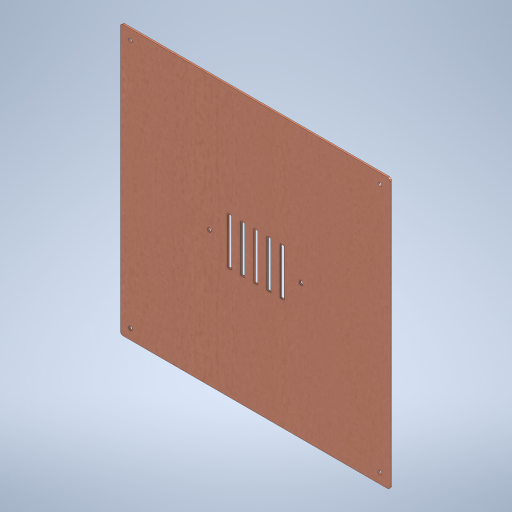
# Autodesk Inventor part: Tapadera
Saved by Autodesk Inventor 2024 (Build 280153000, 153)
## iProperties
Created: 2024-07-17
Part Number: Tapadera
Material: Genérico
Document SubType Name: Modeling
Designer: sergi
Density: 1 g/cm^3
Appearance: Valor por defecto
Author: sergi
Autodesk Inventor part; units mm, degrees
ref_plane "YZ Plane" through (0, 0, 0) normal (1, 0, 0) x (0, 1, 0)
ref_plane "XZ Plane" through (0, 0, 0) normal (0, 1, 0) x (-1, 0, 0)
ref_plane "XY Plane" through (0, 0, 0) normal (0, 0, 1) x (1, 0, 0)
sketch "Boceto1" plane through (0, 0, 0) normal (0, 0, 1) x (1, 0, 0)
  line L0 (-198, 0) -> (0, 0) projected
  line L1 (-198, 0) -> (-198, -2) projected
  line L2 (0, -2) -> (-198, -2) projected
  line L3 (0, 0) -> (0, -2) projected
  line L4 (0, -2) -> (0, -200) projected
  line L5 (0, -2) -> (-2, -2) projected
  line L6 (-2, -200) -> (-2, -2) projected
  line L7 (0, -200) -> (-2, -200) projected
  line L8 (-2, -200) -> (-200, -200) projected
  line L9 (-2, -200) -> (-2, -198) projected
  line L10 (-200, -198) -> (-2, -198) projected
  line L11 (-200, -200) -> (-200, -198) projected
  line L12 (-200, -198) -> (-200, 0) projected
  line L13 (-200, -198) -> (-198, -198) projected
  line L14 (-198, 0) -> (-198, -198) projected
  line L15 (-200, 0) -> (-198, 0) projected
  line L16 (0, 0) -> (0, 1.6)
  line L17 (0, 1.6) -> (1.6, 1.6)
  line L18 (1.6, 1.6) -> (-201.6, 1.6)
  line L19 (-201.6, 1.6) -> (-201.6, -201.6)
  line L20 (-201.6, -201.6) -> (1.6, -201.6)
  line L21 (1.6, -201.6) -> (1.6, 1.6)
  line L22 (-203, 1) -> (-203, -201) projected
  line L23 (-201, -203) -> (1, -203) projected
  line L24 (3, -201) -> (3, 1) projected
  line L25 (1, 3) -> (-201, 3) projected
  line L26 (-192.75, -7.25) -> (-7.25, -7.25) projected
  line L27 (-7.25, -7.25) -> (-7.25, -192.75) projected
  line L28 (-7.25, -192.75) -> (-192.75, -192.75) projected
  line L29 (-192.75, -192.75) -> (-192.75, -7.25) projected
  circle A0 centre (-195.25, -4.75) radius 2.1 projected
  circle A1 centre (-4.75, -4.75) radius 2.1 projected
  circle A2 centre (-4.75, -195.25) radius 2.1 projected
  circle A3 centre (-195.25, -195.25) radius 2.1 projected
  arc A4 (-201, 3) -> (-203, 1) centre (-201, 1) ccw projected
  arc A5 (-203, -201) -> (-201, -203) centre (-201, -201) ccw projected
  arc A6 (1, -203) -> (3, -201) centre (1, -201) ccw projected
  arc A7 (3, 1) -> (1, 3) centre (1, 1) ccw projected
  dimension "d0" = 1.6
  dimension "d1" = 1.6
  dimension "d2" = 203.2
  dimension "d3" = 203.2
  constraints: 12 end point, 2 parallel, 2 perpendicular, 1 horizontal, 1 point on line
  measures "d0" distance of L0.end L16.end
  measures "d1" distance of L16.end L17.end
  measures "d2" distance of L20.end L19.end
  measures "d3" distance of L19.end L18.end
extrude "Extrusión1" add sketch "Boceto1" along normal blind 1.2 contours L17 L21 L20 L19 L18 | L0 L3 L2 L1 | L1 L14 L10 L12 L15 | L2 L6 L10 L14 | L4 L7 L6 L2 | L10 L6 L8 L11 | A4 L25 A7 L24 A6 L23 A5 L22 | L26 L27 L28 L29 | A0 | A1 | A2 | A3
sketch "Boceto2" plane through (0, 0, 1.2) normal (0, 0, 1) x (1, 0, 0)
  line L0 (-192.75, -7.25) -> (-7.25, -7.25) projected
  line L1 (-7.25, -7.25) -> (-7.25, -192.75) projected
  line L2 (-2.25, -197.75) -> (-2.25, -2.25) projected
  line L3 (-2.25, -2.25) -> (-197.75, -2.25) projected
  line L4 (-7.25, -7.25) -> (-2.25, -2.25)
  circle A0 centre (-4.75, -4.75) radius 1.5
  line L5 (-201, -203) -> (1, -203) projected
  line L6 (-203, -203) -> (-203, -195.25)
  line L7 (-203, 1) -> (-203, -201) projected
  line L8 (-203, -195.25) -> (-195.25, -195.25)
  circle A1 centre (-195.25, -195.25) radius 1.5
  line L9 (3, -203) -> (-4.75, -203)
  line L10 (-4.75, -203) -> (-4.75, -195.25)
  circle A2 centre (-4.75, -195.25) radius 1.5
  line L11 (-203, 3) -> (-195.25, 3)
  line L12 (1, 3) -> (-201, 3) projected
  line L13 (-195.25, 3) -> (-195.25, -4.75)
  circle A3 centre (-195.25, -4.75) radius 1.5
  point P0 (0, 0)
  point P1 (3, 3)
  dimension "d6" = 3
  dimension "d14" = 7.75
  dimension "d15" = 7.75
  dimension "d16" = 3
  dimension "d17" = 7.75
  dimension "d18" = 7.75
  dimension "d19" = 3
  dimension "d20" = 7.75
  dimension "d21" = 7.75
  dimension "d22" = 90
  dimension "d23" = 3
  constraints: 14 end point, 4 centre point, 3 coincident, 3 perpendicular, 3 point on line, 1 midpoint
  measures "d6" diameter of A0
  measures "d14" distance of L6.start L6.end
  measures "d15" distance of L6.end L8.end
  measures "d16" diameter of A1
  measures "d17" distance of L9.start L9.end
  measures "d18" distance of L9.end L10.end
  measures "d19" diameter of A2
  measures "d20" distance of L11.start L11.end
  measures "d21" distance of L11.end L13.end
  measures "d22" angle of L11 L13
  measures "d23" diameter of A3
hole "Agujero1" at (-4.75, -4.75, 1.2) at (-195.25, -4.75, 1.2) at (-195.25, -195.25, 1.2) at (-4.75, -195.25, 1.2) direction (0, 0, -1) diameter 3 depth 4
sketch "Boceto3" plane through (0, 0, 1.2) normal (0, 0, 1) x (1, 0, 0)
  line L0 (-125, -122.5) -> (-75, -122.5) projected
  arc A0 (-75, -122.5) -> (-70, -117.5) centre (-75, -117.5) ccw projected
  line L1 (-70, -117.5) -> (-70, -112.2474) projected
  arc A1 (-64, -104.899) -> (-70, -112.2474) centre (-62.5, -112.2474) ccw projected
  arc A2 (-64, -104.899) -> (-64, -95.101) centre (-65, -100) ccw projected
  arc A3 (-70, -87.7526) -> (-64, -95.101) centre (-62.5, -87.7526) ccw projected
  line L2 (-70, -87.7526) -> (-70, -82.5) projected
  arc A4 (-70, -82.5) -> (-75, -77.5) centre (-75, -82.5) ccw projected
  line L3 (-75, -77.5) -> (-125, -77.5) projected
  arc A5 (-125, -77.5) -> (-130, -82.5) centre (-125, -82.5) ccw projected
  line L4 (-130, -82.5) -> (-130, -87.7526) projected
  arc A6 (-136, -95.101) -> (-130, -87.7526) centre (-137.5, -87.7526) ccw projected
  arc A7 (-136, -95.101) -> (-136, -104.899) centre (-135, -100) ccw projected
  arc A8 (-130, -112.2474) -> (-136, -104.899) centre (-137.5, -112.2474) ccw projected
  line L5 (-130, -112.2474) -> (-130, -117.5) projected
  arc A9 (-130, -117.5) -> (-125, -122.5) centre (-125, -117.5) ccw projected
  line L6 (-125, -121.5) -> (-75, -121.5) projected
  arc A10 (-75, -121.5) -> (-71, -117.5) centre (-75, -117.5) ccw projected
  line L7 (-71, -117.5) -> (-71, -82.5) projected
  arc A11 (-71, -82.5) -> (-75, -78.5) centre (-75, -82.5) ccw projected
  line L8 (-75, -78.5) -> (-125, -78.5) projected
  arc A12 (-125, -78.5) -> (-129, -82.5) centre (-125, -82.5) ccw projected
  line L9 (-129, -82.5) -> (-129, -117.5) projected
  arc A13 (-129, -117.5) -> (-125, -121.5) centre (-125, -117.5) ccw projected
  line L10 (-75, -118) -> (-125, -118)
  arc A14 (-125.5, -117.5) -> (-125, -118) centre (-125, -117.5) ccw
  line L11 (-125.5, -117.5) -> (-125.5, -82.5)
  arc A15 (-125, -82) -> (-125.5, -82.5) centre (-125, -82.5) ccw
  line L12 (-125, -82) -> (-75, -82)
  arc A16 (-74.5, -82.5) -> (-75, -82) centre (-75, -82.5) ccw
  line L13 (-74.5, -82.5) -> (-74.5, -117.5)
  arc A17 (-75, -118) -> (-74.5, -117.5) centre (-75, -117.5) ccw
  line L14 (-74.5, -118) -> (-74.5, -82)
  line L15 (-78, -118) -> (-78, -82)
  line L16 (-81, -118) -> (-81, -82)
  line L17 (-88, -118) -> (-88, -82)
  line L18 (-91, -118) -> (-91, -82)
  line L19 (-98, -118) -> (-98, -82)
  line L20 (-101, -118) -> (-101, -82)
  line L21 (-108, -118) -> (-108, -82)
  line L22 (-111, -118) -> (-111, -82)
  line L23 (-118, -118) -> (-118, -82)
  line L24 (-121, -118) -> (-121, -82)
  circle A18 centre (-65, -100) radius 1.5
  circle A19 centre (-135, -100) radius 1.5
  point P0 (0, 0)
  dimension "d24" = 3.5
  dimension "d25" = 3
  dimension "d26" = 7
  dimension "d27" = 3
  dimension "d28" = 7
  dimension "d29" = 3
  dimension "d30" = 7
  dimension "d31" = 3
  dimension "d32" = 7
  dimension "d33" = 3
  dimension "d36" = 3
  dimension "d37" = 3
  constraints: 30 end point, 10 parallel, 8 point on circle, 6 centre point, 2 coincident, 1 point on line, 7 other
  measures "d24" distance between parallel lines of L14 L15
  measures "d25" distance between parallel lines of L15 L16
  measures "d26" distance between parallel lines of L16 L17
  measures "d27" distance between parallel lines of L17 L18
  measures "d28" distance between parallel lines of L18 L19
  measures "d29" distance between parallel lines of L19 L20
  measures "d30" distance between parallel lines of L20 L21
  measures "d31" distance between parallel lines of L21 L22
  measures "d32" distance between parallel lines of L22 L23
  measures "d33" distance between parallel lines of L23 L24
  measures "d36" diameter of A18
  measures "d37" diameter of A19
extrude "Extrusión2" cut sketch "Boceto3" against normal blind 3 contours L10 L16 L12 L15 | L10 L18 L12 L17 | L10 L20 L12 L19 | L10 L22 L12 L21 | L10 L24 L12 L23 | A18 | A19
